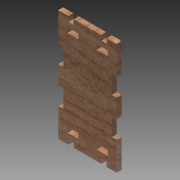
# Autodesk Inventor part: holder_ceil_plate
Saved by Autodesk Inventor 2014 SP1 (Build 180222100, 222)
## iProperties
Created: 2014-01-06
Part Number: holder_ceil_plate
Material: Wood (Birch)
Document SubType Name: Modeling
Designer: aoki
Density: 1 g/cm^3
Appearance: Birch - Natural Polished
Author: aoki
Autodesk Inventor part; units mm, degrees
ref_plane "YZ Plane" through (0, 0, 0) normal (1, 0, 0) x (0, 1, 0)
ref_plane "XZ Plane" through (0, 0, 0) normal (0, 1, 0) x (-1, 0, 0)
ref_plane "XY Plane" through (0, 0, 0) normal (0, 0, 1) x (1, 0, 0)
sketch "Block1" plane through (0, 0, 0) normal (0, 0, 1) x (1, 0, 0)
  line L0 (-15.1, 61.1) -> (15.1, 61.1)
  line L1 (15.1, 61.1) -> (15.1, 52.1)
  line L2 (15.1, 52.1) -> (20.9, 52.1)
  line L3 (20.9, 52.1) -> (20.9, 61.1)
  line L4 (20.9, 61.1) -> (35.6, 61.1)
  line L5 (35.6, 61.1) -> (35.6, 29.9)
  line L6 (35.6, 29.9) -> (26.6, 29.9)
  line L7 (26.6, 29.9) -> (26.6, 10.1)
  line L8 (26.6, 10.1) -> (35.6, 10.1)
  line L9 (35.6, 10.1) -> (35.6, -10.1)
  line L10 (35.6, -10.1) -> (26.6, -10.1)
  line L11 (26.6, -10.1) -> (26.6, -29.9)
  line L12 (26.6, -29.9) -> (35.6, -29.9)
  line L13 (35.6, -29.9) -> (35.6, -61.1)
  line L14 (35.6, -61.1) -> (20.9, -61.1)
  line L15 (20.9, -61.1) -> (20.9, -52.1)
  line L16 (20.9, -52.1) -> (15.1, -52.1)
  line L17 (15.1, -52.1) -> (15.1, -61.1)
  line L18 (15.1, -61.1) -> (-15.1, -61.1)
  line L19 (-15.1, -61.1) -> (-15.1, -52.1)
  line L20 (-15.1, -52.1) -> (-20.9, -52.1)
  line L21 (-20.9, -52.1) -> (-20.9, -61.1)
  line L22 (-20.9, -61.1) -> (-35.6, -61.1)
  line L23 (-35.6, -61.1) -> (-35.6, -29.9)
  line L24 (-35.6, -29.9) -> (-26.6, -29.9)
  line L25 (-26.6, -29.9) -> (-26.6, -10.1)
  line L26 (-26.6, -10.1) -> (-35.6, -10.1)
  line L27 (-35.6, -10.1) -> (-35.6, 10.1)
  line L28 (-35.6, 10.1) -> (-26.6, 10.1)
  line L29 (-26.6, 10.1) -> (-26.6, 29.9)
  line L30 (-26.6, 29.9) -> (-35.6, 29.9)
  line L31 (-35.6, 29.9) -> (-35.6, 61.1)
  line L32 (-35.6, 61.1) -> (-20.9, 61.1)
  line L33 (-20.9, 61.1) -> (-20.9, 52.1)
  line L34 (-20.9, 52.1) -> (-15.1, 52.1)
  line L35 (-15.1, 52.1) -> (-15.1, 61.1)
  line L36 (-9.9, 50.1) -> (-22.1, 50.1)
  line L37 (-22.1, 50.1) -> (-22.1, 40.9)
  line L38 (-22.1, 40.9) -> (-9.9, 40.9)
  line L39 (-9.9, 40.9) -> (-9.9, 50.1)
  line L40 (22.1, 50.1) -> (22.1, 40.9)
  line L41 (22.1, 40.9) -> (9.9, 40.9)
  line L42 (9.9, 40.9) -> (9.9, 50.1)
  line L43 (9.9, 50.1) -> (22.1, 50.1)
  line L44 (22.1, -40.9) -> (9.9, -40.9)
  line L45 (9.9, -40.9) -> (9.9, -50.1)
  line L46 (9.9, -50.1) -> (22.1, -50.1)
  line L47 (22.1, -50.1) -> (22.1, -40.9)
  line L48 (-9.9, -40.9) -> (-22.1, -40.9)
  line L49 (-22.1, -40.9) -> (-22.1, -50.1)
  line L50 (-22.1, -50.1) -> (-9.9, -50.1)
  line L51 (-9.9, -50.1) -> (-9.9, -40.9)
  point P0 (0, 0)
sketch "Block2" plane through (0, 0, 0) normal (0, 0, 1) x (1, 0, 0)
  line L0 (20.8, 61.2) -> (35.7, 61.2)
  line L1 (35.7, 61.2) -> (35.7, 29.8)
  line L2 (35.7, 29.8) -> (26.7, 29.8)
  line L3 (26.7, 29.8) -> (26.7, 10.2)
  line L4 (26.7, 10.2) -> (35.7, 10.2)
  line L5 (35.7, 10.2) -> (35.7, -10.2)
  line L6 (35.7, -10.2) -> (26.7, -10.2)
  line L7 (26.7, -10.2) -> (26.7, -29.8)
  line L8 (26.7, -29.8) -> (35.7, -29.8)
  line L9 (35.7, -29.8) -> (35.7, -61.2)
  line L10 (35.7, -61.2) -> (20.8, -61.2)
  line L11 (20.8, -61.2) -> (20.8, -52.2)
  line L12 (20.8, -52.2) -> (15.2, -52.2)
  line L13 (15.2, -52.2) -> (15.2, -61.2)
  line L14 (15.2, -61.2) -> (-15.2, -61.2)
  line L15 (-15.2, -61.2) -> (-15.2, -52.2)
  line L16 (-15.2, -52.2) -> (-20.8, -52.2)
  line L17 (-20.8, -52.2) -> (-20.8, -61.2)
  line L18 (-20.8, -61.2) -> (-35.7, -61.2)
  line L19 (-35.7, -61.2) -> (-35.7, -29.8)
  line L20 (-35.7, -29.8) -> (-26.7, -29.8)
  line L21 (-26.7, -29.8) -> (-26.7, -10.2)
  line L22 (-26.7, -10.2) -> (-35.7, -10.2)
  line L23 (-35.7, -10.2) -> (-35.7, 10.2)
  line L24 (-35.7, 10.2) -> (-26.7, 10.2)
  line L25 (-26.7, 10.2) -> (-26.7, 29.8)
  line L26 (-26.7, 29.8) -> (-35.7, 29.8)
  line L27 (-35.7, 29.8) -> (-35.7, 61.2)
  line L28 (-35.7, 61.2) -> (-20.8, 61.2)
  line L29 (-20.8, 61.2) -> (-20.8, 52.2)
  line L30 (-20.8, 52.2) -> (-15.2, 52.2)
  line L31 (-15.2, 52.2) -> (-15.2, 61.2)
  line L32 (-15.2, 61.2) -> (15.2, 61.2)
  line L33 (15.2, 61.2) -> (15.2, 52.2)
  line L34 (15.2, 52.2) -> (20.8, 52.2)
  line L35 (20.8, 52.2) -> (20.8, 61.2)
  line L36 (22.2, 50.2) -> (22.2, 40.8)
  line L37 (22.2, 40.8) -> (9.8, 40.8)
  line L38 (9.8, 40.8) -> (9.8, 50.2)
  line L39 (9.8, 50.2) -> (22.2, 50.2)
  line L40 (-9.8, 50.2) -> (-22.2, 50.2)
  line L41 (-22.2, 50.2) -> (-22.2, 40.8)
  line L42 (-22.2, 40.8) -> (-9.8, 40.8)
  line L43 (-9.8, 40.8) -> (-9.8, 50.2)
  line L44 (-9.8, -40.8) -> (-22.2, -40.8)
  line L45 (-22.2, -40.8) -> (-22.2, -50.2)
  line L46 (-22.2, -50.2) -> (-9.8, -50.2)
  line L47 (-9.8, -50.2) -> (-9.8, -40.8)
  line L48 (22.2, -40.8) -> (9.8, -40.8)
  line L49 (9.8, -40.8) -> (9.8, -50.2)
  line L50 (9.8, -50.2) -> (22.2, -50.2)
  line L51 (22.2, -50.2) -> (22.2, -40.8)
  point P0 (0, 0)
sketch "Block3" plane through (0, 0, 0) normal (0, 0, 1) x (1, 0, 0)
  line L0 (20.9, 61.1) -> (35.6, 61.1)
  line L1 (35.6, 61.1) -> (35.6, 29.9)
  line L2 (35.6, 29.9) -> (26.6, 29.9)
  line L3 (26.6, 29.9) -> (26.6, 10.1)
  line L4 (26.6, 10.1) -> (35.6, 10.1)
  line L5 (35.6, 10.1) -> (35.6, -10.1)
  line L6 (35.6, -10.1) -> (26.6, -10.1)
  line L7 (26.6, -10.1) -> (26.6, -29.9)
  line L8 (26.6, -29.9) -> (35.6, -29.9)
  line L9 (35.6, -29.9) -> (35.6, -61.1)
  line L10 (35.6, -61.1) -> (20.9, -61.1)
  line L11 (20.9, -61.1) -> (20.9, -52.1)
  line L12 (20.9, -52.1) -> (15.1, -52.1)
  line L13 (15.1, -52.1) -> (15.1, -61.1)
  line L14 (15.1, -61.1) -> (-15.1, -61.1)
  line L15 (-15.1, -61.1) -> (-15.1, -52.1)
  line L16 (-15.1, -52.1) -> (-20.9, -52.1)
  line L17 (-20.9, -52.1) -> (-20.9, -61.1)
  line L18 (-20.9, -61.1) -> (-35.6, -61.1)
  line L19 (-35.6, -61.1) -> (-35.6, -29.9)
  line L20 (-35.6, -29.9) -> (-26.6, -29.9)
  line L21 (-26.6, -29.9) -> (-26.6, -10.1)
  line L22 (-26.6, -10.1) -> (-35.6, -10.1)
  line L23 (-35.6, -10.1) -> (-35.6, 10.1)
  line L24 (-35.6, 10.1) -> (-26.6, 10.1)
  line L25 (-26.6, 10.1) -> (-26.6, 29.9)
  line L26 (-26.6, 29.9) -> (-35.6, 29.9)
  line L27 (-35.6, 29.9) -> (-35.6, 61.1)
  line L28 (-35.6, 61.1) -> (-20.9, 61.1)
  line L29 (-20.9, 61.1) -> (-20.9, 52.1)
  line L30 (-20.9, 52.1) -> (-15.1, 52.1)
  line L31 (-15.1, 52.1) -> (-15.1, 61.1)
  line L32 (-15.1, 61.1) -> (15.1, 61.1)
  line L33 (15.1, 61.1) -> (15.1, 52.1)
  line L34 (15.1, 52.1) -> (20.9, 52.1)
  line L35 (20.9, 52.1) -> (20.9, 61.1)
  line L36 (22.1, 50.1) -> (22.1, 40.9)
  line L37 (22.1, 40.9) -> (9.9, 40.9)
  line L38 (9.9, 40.9) -> (9.9, 50.1)
  line L39 (9.9, 50.1) -> (22.1, 50.1)
  line L40 (-9.9, 50.1) -> (-22.1, 50.1)
  line L41 (-22.1, 50.1) -> (-22.1, 40.9)
  line L42 (-22.1, 40.9) -> (-9.9, 40.9)
  line L43 (-9.9, 40.9) -> (-9.9, 50.1)
  line L44 (-9.9, -40.9) -> (-22.1, -40.9)
  line L45 (-22.1, -40.9) -> (-22.1, -50.1)
  line L46 (-22.1, -50.1) -> (-9.9, -50.1)
  line L47 (-9.9, -50.1) -> (-9.9, -40.9)
  line L48 (22.1, -40.9) -> (9.9, -40.9)
  line L49 (9.9, -40.9) -> (9.9, -50.1)
  line L50 (9.9, -50.1) -> (22.1, -50.1)
  line L51 (22.1, -50.1) -> (22.1, -40.9)
  point P0 (0, 0)
sketch "Block4" plane through (0, 0, 0) normal (0, 0, 1) x (1, 0, 0)
  line L0 (-15.08, 61.08) -> (15.08, 61.08)
  line L1 (15.08, 61.08) -> (15.08, 55.58)
  line L2 (15.08, 55.58) -> (20.92, 55.58)
  line L3 (20.92, 55.58) -> (20.92, 61.08)
  line L4 (20.92, 61.08) -> (32.08, 61.08)
  line L5 (32.08, 61.08) -> (32.08, 29.92)
  line L6 (32.08, 29.92) -> (26.58, 29.92)
  line L7 (26.58, 29.92) -> (26.58, 10.08)
  line L8 (26.58, 10.08) -> (32.08, 10.08)
  line L9 (32.08, 10.08) -> (32.08, -10.08)
  line L10 (32.08, -10.08) -> (26.58, -10.08)
  line L11 (26.58, -10.08) -> (26.58, -29.92)
  line L12 (26.58, -29.92) -> (32.08, -29.92)
  line L13 (32.08, -29.92) -> (32.08, -61.08)
  line L14 (32.08, -61.08) -> (20.92, -61.08)
  line L15 (20.92, -61.08) -> (20.92, -55.58)
  line L16 (20.92, -55.58) -> (15.08, -55.58)
  line L17 (15.08, -55.58) -> (15.08, -61.08)
  line L18 (15.08, -61.08) -> (-15.08, -61.08)
  line L19 (-15.08, -61.08) -> (-15.08, -55.58)
  line L20 (-15.08, -55.58) -> (-20.92, -55.58)
  line L21 (-20.92, -55.58) -> (-20.92, -61.08)
  line L22 (-20.92, -61.08) -> (-32.08, -61.08)
  line L23 (-32.08, -61.08) -> (-32.08, -29.92)
  line L24 (-32.08, -29.92) -> (-26.58, -29.92)
  line L25 (-26.58, -29.92) -> (-26.58, -10.08)
  line L26 (-26.58, -10.08) -> (-32.08, -10.08)
  line L27 (-32.08, -10.08) -> (-32.08, 10.08)
  line L28 (-32.08, 10.08) -> (-26.58, 10.08)
  line L29 (-26.58, 10.08) -> (-26.58, 29.92)
  line L30 (-26.58, 29.92) -> (-32.08, 29.92)
  line L31 (-32.08, 29.92) -> (-32.08, 61.08)
  line L32 (-32.08, 61.08) -> (-20.92, 61.08)
  line L33 (-20.92, 61.08) -> (-20.92, 55.58)
  line L34 (-20.92, 55.58) -> (-15.08, 55.58)
  line L35 (-15.08, 55.58) -> (-15.08, 61.08)
  line L36 (-9.92, 50.08) -> (-22.08, 50.08)
  line L37 (-22.08, 50.08) -> (-22.08, 44.42)
  line L38 (-22.08, 44.42) -> (-9.92, 44.42)
  line L39 (-9.92, 44.42) -> (-9.92, 50.08)
  line L40 (22.08, 50.08) -> (22.08, 44.42)
  line L41 (22.08, 44.42) -> (9.92, 44.42)
  line L42 (9.92, 44.42) -> (9.92, 50.08)
  line L43 (9.92, 50.08) -> (22.08, 50.08)
  line L44 (-9.92, -44.42) -> (-22.08, -44.42)
  line L45 (-22.08, -44.42) -> (-22.08, -50.08)
  line L46 (-22.08, -50.08) -> (-9.92, -50.08)
  line L47 (-9.92, -50.08) -> (-9.92, -44.42)
  line L48 (22.08, -44.42) -> (9.92, -44.42)
  line L49 (9.92, -44.42) -> (9.92, -50.08)
  line L50 (9.92, -50.08) -> (22.08, -50.08)
  line L51 (22.08, -50.08) -> (22.08, -44.42)
  point P0 (0, 0)
sketch "Sketch1" plane through (0, 0, 0) normal (0, 1, 0) x (-1, 0, 0)
  line L0 (32, -50) -> (-32, -50)
  line L1 (-32, -50) -> (-32, 50)
  line L2 (-32, 50) -> (32, 50)
  line L3 (32, 50) -> (32, -50)
  line L4 (32, -50) -> (-32, 50) construction
  line L5 (-32, -50) -> (32, 50) construction
  point P0 (0, 0)
  dimension "d0" = 64
  dimension "d1" = 100
  constraints: 12 end point, 2 midpoint, 2 parallel, 1 horizontal, 1 perpendicular
  measures "d0" distance of L1.end L2.end
  measures "d1" distance of L0.end L1.end
extrude "Extrusion1" add sketch "Sketch1" along normal blind 5.5
sketch "Sketch5" plane through (0, 5.5, 0) normal (0, 1, 0) x (1, 0, 0)
  line L0 (32, 50) -> (-32, 50) projected
  line L1 (-32, 50) -> (-32, -50) projected
  line L2 (-32, 30) -> (-26.5, 30)
  line L3 (-26.5, 30) -> (-26.5, 10)
  line L4 (-26.5, 10) -> (-32, 10)
  line L5 (-32, 10) -> (-32, 30)
  line L6 (-66.327, 0) -> (148.7623, 0) projected
  line L7 (0, 85.6282) -> (0, -86.069) projected
  line L8 (-32, -30) -> (-26.5, -30)
  line L9 (-26.5, -30) -> (-26.5, -10)
  line L10 (-26.5, -10) -> (-32, -10)
  line L11 (-32, -10) -> (-32, -30)
  line L12 (32, 30) -> (26.5, 30)
  line L13 (26.5, 30) -> (26.5, 10)
  line L14 (26.5, 10) -> (32, 10)
  line L15 (32, 10) -> (32, 30)
  line L16 (32, -30) -> (26.5, -30)
  line L17 (26.5, -30) -> (26.5, -10)
  line L18 (26.5, -10) -> (32, -10)
  line L19 (32, -10) -> (32, -30)
  point P0 (0, 0)
  dimension "d12" = 20
  dimension "d13" = 20
  dimension "d14" = 5.5
  constraints: 32 end point, 12 symmetric about line, 2 parallel, 1 collinear, 1 horizontal, 1 perpendicular
  measures "d12" distance between parallel lines of L0 L2
  measures "d13" distance of L2.end L3.end
  measures "d14" distance of L3.end L4.end
extrude "Extrusion3" cut sketch "Sketch5" against normal through all contours L2 L3 L4 L1 | L10 L9 L8 L1 | L15 L14 L13 L12 | L16 L17 L18 L19
sketch "Sketch6" plane through (0, 5.5, 0) normal (0, 1, 0) x (1, 0, 0)
  line L0 (32, 50) -> (-32, 50) projected
  line L1 (-66.327, 0) -> (148.7623, 0) projected
  line L2 (0, 85.6282) -> (0, -86.069) projected
  line L3 (-22, 50) -> (-10, 50)
  line L4 (-10, 50) -> (-10, 44.5)
  line L5 (-10, 44.5) -> (-22, 44.5)
  line L6 (-22, 44.5) -> (-22, 50)
  line L7 (22, 50) -> (10, 50)
  line L8 (10, 50) -> (10, 44.5)
  line L9 (10, 44.5) -> (22, 44.5)
  line L10 (22, 44.5) -> (22, 50)
  line L11 (-22, -50) -> (-10, -50)
  line L12 (-10, -50) -> (-10, -44.5)
  line L13 (-10, -44.5) -> (-22, -44.5)
  line L14 (-22, -44.5) -> (-22, -50)
  line L15 (10, -44.5) -> (22, -44.5)
  line L16 (22, -50) -> (10, -50)
  line L17 (10, -50) -> (10, -44.5)
  line L18 (22, -44.5) -> (22, -50)
  point P0 (0, 0)
  dimension "d17" = 5.5
  dimension "d18" = 12
  dimension "d19" = 20
  constraints: 32 end point, 12 symmetric about line, 2 parallel, 1 horizontal, 1 perpendicular, 1 point on line
  measures "d17" distance of L3.end L4.end
  measures "d18" distance of L4.end L5.end
  measures "d19" distance between parallel lines of L8 L4
extrude "Extrusion4" cut sketch "Sketch6" against normal through all
sketch "Sketch7" plane through (0, 0, 0) normal (0, -1, 0) x (1, 0, 0)
  line L0 (-32, -50) -> (32, -50)
  line L1 (32, -50) -> (32, -61)
  line L2 (32, -61) -> (-32, -61)
  line L3 (-32, -61) -> (-32, -50)
  line L4 (-66.327, 0) -> (148.7623, 0) projected
  line L5 (0, -85.6282) -> (0, 86.069) projected
  line L6 (-15, -61) -> (-21, -61)
  line L7 (-21, -61) -> (-21, -55.5)
  line L8 (-21, -55.5) -> (-15, -55.5)
  line L9 (-15, -55.5) -> (-15, -61)
  line L10 (15, -61) -> (21, -61)
  line L11 (21, -61) -> (21, -55.5)
  line L12 (21, -55.5) -> (15, -55.5)
  line L13 (15, -55.5) -> (15, -61)
  line L14 (-32, 50) -> (32, 50)
  line L15 (32, 50) -> (32, 61)
  line L16 (32, 61) -> (-32, 61)
  line L17 (-32, 61) -> (-32, 50)
  line L18 (-32, 50) -> (-22, 50)
  line L19 (-10, 50) -> (10, 50)
  line L20 (22, 50) -> (32, 50)
  line L21 (-15, 61) -> (-21, 61)
  line L22 (-21, 61) -> (-21, 55.5)
  line L23 (-21, 55.5) -> (-15, 55.5)
  line L24 (-15, 55.5) -> (-15, 61)
  line L25 (21, 55.5) -> (15, 55.5)
  line L26 (15, 55.5) -> (15, 61)
  line L27 (15, 61) -> (21, 61)
  line L28 (21, 61) -> (21, 55.5)
  point P0 (0, 0)
  point P1 (32, -50)
  dimension "d22" = 11
  dimension "d23" = 6
  dimension "d24" = 5.5
  dimension "d32" = 15
  dimension "d55" = 64
  constraints: 54 end point, 16 symmetric about line, 4 parallel, 2 horizontal, 2 perpendicular, 1 point on line
  measures "d22" distance of L0.end L1.end
  measures "d23" distance of L7.end L8.end
  measures "d24" distance of L8.end L6.start
  measures "d32" distance between parallel lines of L9 L5
  measures "d55" distance of L16.start L16.end
extrude "Extrusion7" add sketch "Sketch7" against normal blind 5.5 contours L0 L5 L2 L9 L8 L7 L3 | L0 L1 L2 L11 L12 L13 L5 | L14 L17 L16 L22 L23 L24 L5 | L5 L16 L26 L25 L28 L15 L14
equation "\"d2\" = Wt"
equation "\"d14\" = Wt"
equation "\"d15\" = Wt"
equation "\"d17\" = Wt"
equation "\"d20\" = Wt"
equation "\"d24\" = Wt"
equation "\"d55\" = d0"
equation "\"d33\" = Wt"
equation "\"Wt\" = 5.5"
body "Solid1"
